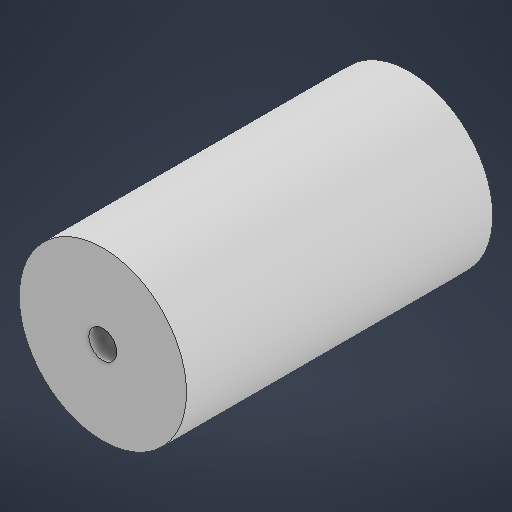
# Autodesk Inventor part: detector holder
Saved by Autodesk Inventor 2026.1 (Build 301233020, 233B)
## iProperties
Created: 2025-12-21
Part Number: detector holder
Material: Ogólny
Document SubType Name: Modeling
Designer: maciej
Density: 1 g/cm^3
Appearance: Domyślna
Author: maciej
Autodesk Inventor part; units mm, degrees
ref_plane "YZ Plane" through (0, 0, 0) normal (1, 0, 0) x (0, 1, 0)
ref_plane "XZ Plane" through (0, 0, 0) normal (0, 1, 0) x (-1, 0, 0)
ref_plane "XY Plane" through (0, 0, 0) normal (0, 0, 1) x (1, 0, 0)
sketch "Sketch1" plane through (0, 0, 0) normal (0, 0, 1) x (1, 0, 0)
  circle A0 centre (0, 0) radius 2.75
  circle A1 centre (0, 0) radius 6
  circle A2 centre (0, 0) radius 1
  circle A3 centre (0, 0) radius 2.25
  circle A4 centre (0, 0) radius 3.25
  dimension "d0" = 5.5
  dimension "d1" = 12
  dimension "d2" = 2
  dimension "d5" = 4.5
  dimension "d6" = 6.5
  constraints: 5 centre point, 5 coincident
  measures "d0" diameter of A0
  measures "d1" diameter of A1
  measures "d2" diameter of A2
  measures "d5" diameter of A3
  measures "d6" diameter of A4
extrude "Extrusion1" add sketch "Sketch1" along normal blind 2 contours A0 | A1 | A3 | A4
extrude "Extrusion2" add sketch "Sketch1" against normal blind 3 contours A0 | A1 | A4
extrude "Extrusion3" add sketch "Sketch1" against normal blind 13 contours A1 | A4
extrude "Extrusion4" add sketch "Sketch1" against normal blind 20 contours A1
body "Solid1"
